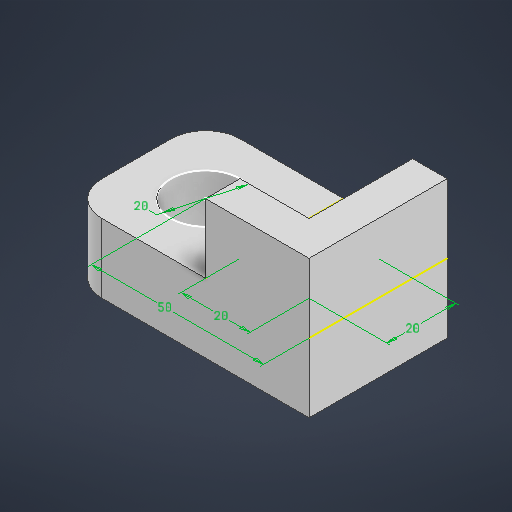
# Autodesk Inventor part: b1
Saved by Autodesk Inventor 2025.4 (Build 294407000, 407)
## iProperties
Created: 2026-05-07
Part Number: b1
Material: Generic
Document SubType Name: Modeling
Designer: VuQuan
Density: 1 g/cm^3
Appearance: Default
Author: VuQuan
Autodesk Inventor part; units mm, degrees
ref_plane "YZ Plane" through (0, 0, 0) normal (1, 0, 0) x (0, 1, 0)
ref_plane "XZ Plane" through (0, 0, 0) normal (0, 1, 0) x (-1, 0, 0)
ref_plane "XY Plane" through (0, 0, 0) normal (0, 0, 1) x (1, 0, 0)
sketch "Sketch1" plane through (0, 0, 0) normal (0, 0, 1) x (1, 0, 0)
  line L0 (0, 0) -> (70, 0)
  line L1 (70, 0) -> (70, 40)
  line L2 (70, 40) -> (40, 40)
  line L3 (40, 40) -> (40, 20)
  line L4 (40, 20) -> (0, 20)
  line L5 (0, 20) -> (0, 0)
  dimension "d0" = 70
  dimension "d1" = 40
  dimension "d2" = 30
  dimension "d3" = 20
  constraints: 12 end point, 3 perpendicular, 2 horizontal, 1 vertical
  measures "d0" distance of L0.start L0.end
  measures "d1" distance of L0.end L1.end
  measures "d2" distance of L1.end L2.end
  measures "d3" distance of L4.end L0.start
extrude "Extrusion1" add sketch "Sketch1" along normal blind 40
sketch "Sketch2" plane through (0, 20, 0) normal (0, 1, 0) x (1, 0, 0)
  line L0 (40, 0) -> (40, -40) projected
  circle A0 centre (20, -20) radius 10
  line L1 (70, 0) -> (70, -40) projected
  line L2 (40, 0) -> (40, -40) projected
  line L3 (40, -10) -> (60, -10)
  line L4 (60, -10) -> (60, -30)
  line L5 (60, -30) -> (40, -30)
  point P0 (40, -20)
  point P1 (60, -20)
  point P2 (40, -20)
  dimension "d6" = 20
  dimension "d7" = 50
  dimension "d8" = 20
  dimension "d9" = 20
  constraints: 6 end point, 3 midpoint, 3 perpendicular, 2 horizontal alignment, 2 point on line, 1 centre point
  measures "d6" diameter of A0
  measures "d7" distance from line of L1 A0.centre
  measures "d8" distance of L4.end L5.end
  measures "d9" distance of L3.end L4.end
extrude "Extrusion2" cut sketch "Sketch2" against normal up to next contours A0
extrude "Extrusion3" cut sketch "Sketch2" along normal through all contours L3 L4 L5 L0
chamfer "Chamfer1" distance 20 angle 45 1 edges at (40, 40, 5)
fillet "Fillet1" radius 10 2 edges at (0, 10, 40) (0, 10, 0)
body "Solid1"
